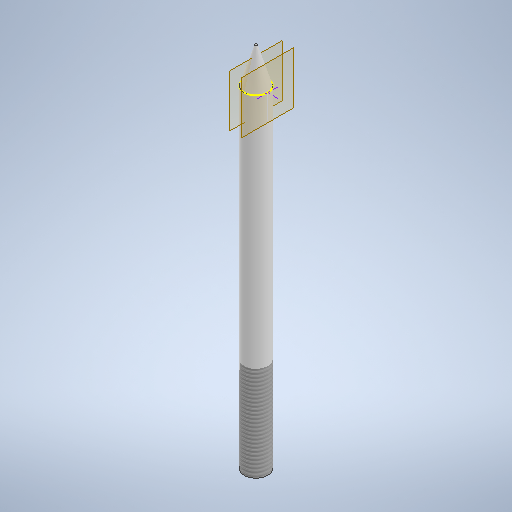
# Autodesk Inventor part: Output link probe
Saved by Autodesk Inventor 2026.3 (Build 303398000, 398)
## iProperties
Created: 2026-07-24
Part Number: Output link probe
Material: Generic
Document SubType Name: Sheet Metal
Designer: matot
Density: 1 g/cm^3
Sheet Metal Rule: Default_mm
Appearance: Default
Author: matot
Autodesk Inventor part; units mm, degrees
ref_plane "YZ Plane" through (0, 0, 0) normal (1, 0, 0) x (0, 1, 0)
ref_plane "XZ Plane" through (0, 0, 0) normal (0, 1, 0) x (-1, 0, 0)
ref_plane "XY Plane" through (0, 0, 0) normal (0, 0, 1) x (1, 0, 0)
sketch "Sketch1" plane through (0, 0, 0) normal (0, 1, 0) x (-1, 0, 0)
  circle A0 centre (0, 0) radius 5
  dimension "d0" = 10
  constraints: 1 centre point, 1 coincident
  measures "d0" diameter of A0
extrude "Extrusion1" add sketch "Sketch1" along normal blind 140
sketch "Sketch2" plane through (0, 140, 0) normal (0, 1, 0) x (1, 0, 0)
  circle A0 centre (0, 0) radius 5 projected
  point P0 (5, 0)
  constraints: 1 horizontal alignment, 1 other
ref_plane "Work Plane2" through (0, 140, 0) normal (1, 0, 0) x (0, 1, 0)
ref_plane "Work Plane1" through (5, 140, 0) normal (1, 0, 0) x (0, 1, 0)
sketch "Sketch3" plane through (0, 140, 0) normal (1, 0, 0) x (0, 1, 0)
  line L0 (15, 0) -> (0, 0)
  line L1 (0, -5) -> (0, 5) projected
  line L2 (15, 0) -> (15, -0.5)
  line L3 (15, -0.5) -> (0, -5)
  arc A0 (15, -0.5) -> (15.5, 0) centre (15, 0) ccw
  line L4 (15, 0) -> (15.5, 0)
  point P0 (-140, 0)
  dimension "d4" = 15
  dimension "d7" = 0.5
  constraints: 8 end point, 2 perpendicular, 2 point on circle, 1 centre point, 1 coincident, 1 horizontal, 1 midpoint
  measures "d4" distance of L0.start L0.end
  measures "d7" distance of L2.end L0.start
revolve "Revolution1" add sketch "Sketch3" angle 360 about axis through (0, 155, 0) along (0, -1, 0) contours L2 L3 L1 L0
sketch "Sketch4" plane through (0, 140, 0) normal (1, 0, 0) x (0, 1, 0)
  line L0 (15, 0.5) -> (15, -0.5) projected
  line L1 (15.5, 0) -> (15, 0)
  arc A0 (15, -0.5) -> (15.5, 0) centre (14.6982, 0.3018) ccw
  point P0 (-140, 0)
  constraints: 3 end point, 2 point on circle, 1 centre point, 1 horizontal
revolve "Revolution2" add sketch "Sketch4" angle 360 about axis through (0, 155.5, 0) along (0, -1, 0)
thread "Thread1" size "M10x1.5" class "6g" standard "ISO Metric profile" length 40 offset 100
equation "\"BendRadius\" = Thickness"
equation "\"BendReliefWidth\" = Thickness"
equation "\"BendReliefDepth\" = 0.5 * Thickness"
equation "\"CornerReliefSize\" = 4 * Thickness"
equation "\"MinimumRemnant\" = 2 * Thickness"
equation "\"TransitionRadius\" = BendRadius"
equation "\"JacobiRadiusSize\" = BendRadius"
equation "\"GapSize\" = Thickness"
equation "\"Thickness\" = 0.5"
body "Solid1"
